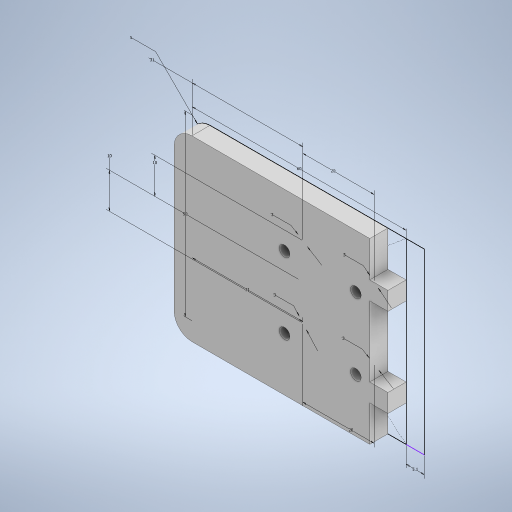
# Autodesk Inventor part: motor chassis holder1
Saved by Autodesk Inventor 2023.2 (Build 272271000, 271)
## iProperties
Created: 2024-08-13
Part Number: motor chassis holder1
Material: Generic
Document SubType Name: Modeling
Designer: PC
Density: 1 g/cm^3
Appearance: Default
Author: PC
Autodesk Inventor part; units mm, degrees
ref_plane "YZ Plane" through (0, 0, 0) normal (1, 0, 0) x (0, 1, 0)
ref_plane "XZ Plane" through (0, 0, 0) normal (0, 1, 0) x (-1, 0, 0)
ref_plane "XY Plane" through (0, 0, 0) normal (0, 0, 1) x (1, 0, 0)
sketch "Sketch1" plane through (0, 0, 0) normal (0, 0, 1) x (1, 0, 0)
  line L0 (30, -25) -> (-25, -25)
  line L1 (-30, -20) -> (-30, 20)
  line L2 (-25, 25) -> (30, 25)
  line L3 (30, 25) -> (30, -25)
  line L4 (30, -25) -> (-30, 25) construction
  line L5 (-30, -25) -> (30, 25) construction
  circle A0 centre (1, -10) radius 1.5
  circle A1 centre (1, 10) radius 1.5
  circle A2 centre (21, 10) radius 1.5
  circle A3 centre (21, -10) radius 1.5
  arc A4 (-25, 25) -> (-30, 20) centre (-25, 20) ccw
  arc A5 (-30, -20) -> (-25, -25) centre (-25, -20) ccw
  line L6 (30, 25) -> (35.1, 25)
  line L7 (35.1, 25) -> (35.1, -25)
  line L8 (35.1, -25) -> (30, -25)
  line L9 (30, -25) -> (30, 25)
  point P0 (0, 0)
  dimension "d0" = 60
  dimension "d1" = 50
  dimension "d2" = 3
  dimension "d3" = 3
  dimension "d4" = 3
  dimension "d5" = 3
  dimension "d6" = 31
  dimension "d7" = 31
  dimension "d8" = 10
  dimension "d9" = 10
  dimension "d10" = 20
  dimension "d11" = 20
  dimension "d12" = 5
  dimension "d13" = 5.1
  constraints: 20 end point, 6 centre point, 4 parallel, 4 point on circle, 4 point on line, 4 tangent, 2 horizontal, 2 horizontal alignment, 2 midpoint, 2 perpendicular, 1 equal radius
  measures "d0" distance of L4.end L2.end
  measures "d1" distance of L5.start L4.end
  measures "d2" diameter of A0
  measures "d3" diameter of A1
  measures "d4" diameter of A2
  measures "d5" diameter of A3
  measures "d6" distance from line of L1 A1.centre
  measures "d7" distance from line of A0.centre L1
  measures "d8" vertical distance of point (0, 0) A1.centre
  measures "d9" vertical distance of point (0, 0) A0.centre
  measures "d10" distance of A2.centre A1.centre
  measures "d11" distance of A3.centre A0.centre
  measures "d12" radius of A4
  measures "d13" distance of L7.end L8.end
extrude "Extrusion1" add sketch "Sketch1" along normal blind 5.1 contours L0 A5 L1 A4 L2 L3
sketch "Sketch3" plane through (0, 0, 5.1) normal (0, 0, 1) x (1, 0, 0)
  line L0 (30, -25) -> (30, 25) projected
  line L1 (30, -9.85) -> (24.9, -9.85)
  line L2 (24.9, -9.85) -> (24.9, 9.85)
  line L3 (24.9, 9.85) -> (30, 9.85)
  line L4 (30, 9.85) -> (30, -9.85)
  line L5 (30, -25) -> (24.9, -25)
  line L6 (24.9, -25) -> (24.9, -14.95)
  line L7 (24.9, -14.95) -> (30, -14.95)
  line L8 (30, -14.95) -> (30, -25)
  line L9 (30, 25) -> (24.9, 25)
  line L10 (24.9, 25) -> (24.9, 14.95)
  line L11 (24.9, 14.95) -> (30, 14.95)
  line L12 (30, 14.95) -> (30, 25)
  point P0 (0, 0)
  point P1 (24.9, 0)
  point P2 (30, 0)
  dimension "d25" = 5.1
  dimension "d26" = 19.7
  dimension "d27" = 5.1
  dimension "d28" = 10.05
  dimension "d29" = 10.05
  constraints: 24 end point, 6 parallel, 3 horizontal, 3 perpendicular, 2 midpoint, 2 point on line, 1 horizontal alignment
  measures "d25" distance of L2.end L3.end
  measures "d26" distance of L1.end L2.end
  measures "d27" distance of L6.end L7.end
  measures "d28" distance of L5.end L6.end
  measures "d29" distance of L10.end L9.end
extrude "Extrusion4" cut sketch "Sketch3" against normal blind 5.1
body "Solid1"
